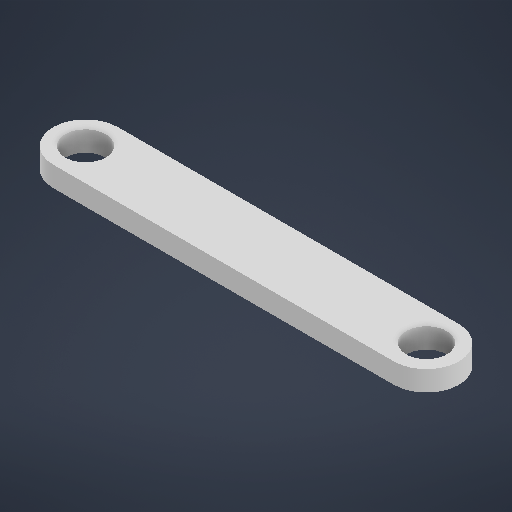
# Autodesk Inventor part: Чертёж
Saved by Autodesk Inventor 2026.2 (Build 302298000, 298)
## iProperties
Created: 2026-02-19
Part Number: Чертёж
Material: Типовые
Document SubType Name: Modeling
Designer: Leonid
Density: 1 g/cm^3
Appearance: По умолчанию
Author: Leonid
Autodesk Inventor part; units mm, degrees
ref_plane "YZ Plane" through (0, 0, 0) normal (1, 0, 0) x (0, 1, 0)
ref_plane "XZ Plane" through (0, 0, 0) normal (0, 1, 0) x (-1, 0, 0)
ref_plane "XY Plane" through (0, 0, 0) normal (0, 0, 1) x (1, 0, 0)
sketch "Эскиз1" plane through (0, 0, 0) normal (0, 1, 0) x (-1, 0, 0)
  line L0 (10.5, 0) -> (-10.5, 0) construction
  line L1 (10.5, 2) -> (-10.5, 2)
  line L2 (-10.5, -2) -> (10.5, -2)
  arc A0 (10.5, -2) -> (10.5, 2) centre (10.5, 0) ccw
  arc A1 (-10.5, 2) -> (-10.5, -2) centre (-10.5, 0) ccw
  circle A2 centre (10.5, 0) radius 1.25
  circle A3 centre (-10.5, 0) radius 1.25
  line L3 (10.5, 5.6569) -> (-10.5, 5.6569) construction
  line L4 (10.5, 7.6569) -> (-10.5, 7.6569)
  line L5 (-10.5, 3.6569) -> (10.5, 3.6569)
  arc A4 (10.5, 3.6569) -> (10.5, 7.6569) centre (10.5, 5.6569) ccw
  arc A5 (-10.5, 7.6569) -> (-10.5, 3.6569) centre (-10.5, 5.6569) ccw
  circle A6 centre (10.5, 5.6569) radius 1.25
  circle A7 centre (-10.5, 5.6569) radius 1.25
  line L6 (10.5, 0) -> (10.5, 5.6569) construction
  point P0 (0, 0)
  point P1 (0, 0)
  point P2 (-12.5, 0)
  point P3 (12.5, 0)
  point P4 (0, 5.6569)
  point P5 (0, 5.6569)
  point P6 (-12.5, 5.6569)
  point P7 (12.5, 5.6569)
  dimension "d0" = 2.5
  dimension "d1" = 2.5
  dimension "d2" = 2
  dimension "d3" = 25
  dimension "d4" = 2.5
  dimension "d5" = 2.5
  dimension "d6" = 2
  dimension "d7" = 25
  dimension "d11" = 5.6569
  dimension "d12" = 90
  constraints: 18 end point, 12 point on circle, 8 centre point, 8 tangent, 6 coincident, 2 horizontal, 2 midpoint, 2 parallel
  measures "d0" diameter of A2
  measures "d1" diameter of A3
  measures "d2" radius of A0
  measures "d3" distance of point (-12.5, 0) point (12.5, 0)
  measures "d4" diameter of A6
  measures "d5" diameter of A7
  measures "d6" radius of A4
  measures "d7" distance of point (-12.5, 5.657) point (12.5, 5.657)
  measures "d11" distance of L6.start L6.end
  measures "d12" angle of L0 L6
extrude "Выдавливание1" add sketch "Эскиз1" along normal blind 1.25 contours A0 L2 A1 L1
